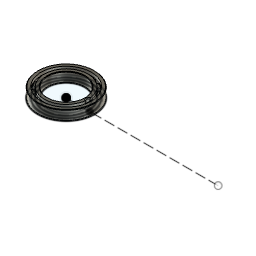
id15 bearing v6 (Autodesk Fusion 360 design; units mm, degrees)
Autodesk Fusion 360 part; units mm, degrees
sketch "Sketch1" plane through (0, 0, 0) normal (0, 0, 1) x (1, 0, 0)
  circle A0 centre (0, 0) radius 7.6
  circle A1 centre (0, 0) radius 8.6 construction
  line L0 (0, 0) -> (62.2874, 0) construction
  circle A2 centre (9.6, 0) radius 1 construction
  circle A3 centre (0, 0) radius 10.6 construction
  circle A4 centre (0, 0) radius 11.6
  circle A5 centre (9.6, 0) radius 0.5 construction
  circle A6 centre (0, 0) radius 9.1
  circle A7 centre (0, 0) radius 10.1
  circle A8 centre (0, 0) radius 8.94
  circle A9 centre (0, 0) radius 10.26
  dimension "d1" = 15.2
  dimension "d2" = 1
  dimension "d3" = 2
  dimension "d4" = 1
  dimension "d5" = 1
  dimension "d6" = -0.16
  dimension "d7" = 0.16
  constraint coincident A0.centre A1.centre
  constraint horizontal L0
  constraint coincident L0 A2.centre
  constraint tangent A1 A2
  constraint concentric A1 A3
  constraint tangent A2 A3
  constraint concentric A0 A4
  constraint concentric A2 A5
  constraint concentric A3 A6
  constraint tangent A5 A6
  constraint concentric A1 A7
  constraint tangent A5 A7
  measures "d1" diameter of A0
  measures "d2" distance of A0 A1
  measures "d3" diameter of A2
  measures "d4" distance of A3 A4
  measures "d5" diameter of A5
extrude "Extrude1" add sketch "Sketch1" along normal blind 4 makes body 1 at (8.9289, -0.4456, 2.6667) makes body 2 at (10.0874, -0.5034, 2.6667) makes body 3 at (11.5856, -0.5782, 2.6667)
sketch "Sketch2" plane through (0, 0, 0) normal (0, 1, 0) x (1, 0, 0)
  line L0 (7.6, 0) -> (7.6, -4) construction
  line L1 (-7.6, -4) -> (-7.6, 0)
  line L2 (9.1, 0) -> (9.1, -4)
  line L3 (-9.1, -4) -> (-9.1, 0)
  line L4 (10.26, 0) -> (10.26, -4) construction
  line L5 (-10.26, -4) -> (-10.26, 0)
  line L6 (8.94, -4) -> (8.94, 0) construction
  line L7 (-8.94, 0) -> (-8.94, -4)
  line L8 (10.1, -4) -> (10.1, 0)
  line L9 (-10.1, 0) -> (-10.1, -4)
  line L10 (11.6, -4) -> (11.6, 0) construction
  line L11 (-11.6, 0) -> (-11.6, -4)
  line L12 (-8.94, -4) -> (-7.6, -4)
  line L13 (7.6, -4) -> (8.94, -4) construction
  line L14 (-10.1, -4) -> (-9.1, -4)
  line L15 (9.1, -4) -> (10.1, -4)
  line L16 (-11.6, -4) -> (-10.26, -4)
  line L17 (10.26, -4) -> (11.6, -4) construction
  line L18 (8.94, 0) -> (7.6, 0) construction
  line L19 (-7.6, 0) -> (-8.94, 0)
  line L20 (10.1, 0) -> (9.1, 0)
  line L21 (-9.1, 0) -> (-10.1, 0)
  line L22 (11.6, 0) -> (10.26, 0) construction
  line L23 (-10.26, 0) -> (-11.6, 0)
  line L24 (7.6, -2) -> (11.6, -2) construction
  line L25 (9.6, -4) -> (9.6, 0) construction
  point P0 (9.6, -2)
  constraint midpoint L0 L24.start
  constraint midpoint L10 L24.end
  constraint midpoint L15 L25.start
  constraint midpoint L20 L25.end
  constraint midpoint L24 P0
sphere "SpherePrimitive1" add diameter 2.1 placed x (1, 0, 0) y (0, 0, -1) z (0, 1, 0) at (9.5, 0, 2) separate body makes body 4
sketch "Sketch5" plane through (0, 0, 0) normal (0, 1, 0) x (1, 0, 0)
  line L0 (-10.1, -4) -> (-9.1, -4)
  line L1 (9.1, -4) -> (10.1, -4)
  line L2 (10.1, 0) -> (9.1, 0)
  line L3 (-9.1, 0) -> (-10.1, 0)
  line L4 (9.1, -4) -> (9.1, 0)
  line L5 (10.1, 0) -> (10.1, -4)
  line L6 (9.6, -4) -> (9.6, 0) construction
  line L7 (9.6, -2) -> (10.1, -2)
  line L8 (9.1, -2.5) -> (10.1, -2.5)
  dimension "d15" = 0.5
  constraint coincident L1.start L4.start
  constraint coincident L2.end L4.end
  constraint coincident L2.start L5.start
  constraint coincident L1.end L5.end
  constraint midpoint L1 L6.start
  constraint midpoint L2 L6.end
  constraint midpoint L6 L7.start
  constraint midpoint L5 L7.end
  constraint coincident L4 L8.start
  constraint coincident L5 L8.end
  constraint perpendicular L5 L8
  measures "d15" distance of L7.start L8
revolve "Revolve2" cut sketch "Sketch5" angle 360 about axis through (0, 0, 1.75) along (0, 0, 1) contours L1 L4 L5 L8 bodies 2
pattern_circular "C-Pattern2" count 15 over 360 about axis through (0, 0, 1.75) along (0, 0, 1) of "SpherePrimitive1" makes body 5 makes body 6 makes body 7 makes body 8 makes body 9 makes body 10 makes body 11 makes body 12 makes body 13 makes body 14 makes body 15 makes body 16 makes body 17 makes body 18
combine "Combine6" operation cut target body 2 tool bodies 4 5 16 17 7 9 6 10 11 8 14 15 12 13 18 keep tools
sketch "Sketch6" plane through (0, 0, 0) normal (0, 1, 0) x (1, 0, 0)
  circle A0 centre (9.5, -2) radius 1.05
  line L0 (8.94, -4) -> (8.94, 0)
  line L1 (-8.94, 0) -> (-8.94, -4)
  line L2 (10.26, 0) -> (10.26, -4)
  line L3 (-10.26, -4) -> (-10.26, 0)
revolve "Revolve3" cut sketch "Sketch6" angle 360 about axis through (0, 0, 1.75) along (0, 0, 1) contours A0 L2 | A0 L0 bodies 1 3
sketch "Sketch7" plane through (0, 0, 2.5) normal (0, 0, 1) x (-1, 0, 0)
  arc A0 (-9.4973, 3.4369) -> (-8.6109, 2.9432) centre (-8.6787, 3.864) ccw
  arc A1 (-9.4973, 3.4369) -> (-10.0741, 0.7231) centre (0, 0) ccw
  arc A2 (-9.0636, 0.8136) -> (-10.0741, 0.7231) centre (-9.5, 0) ccw
  arc A3 (-8.6109, 2.9432) -> (-9.0636, 0.8136) centre (0, 0) ccw
  circle A4 centre (0, 0) radius 10.1
  circle A5 centre (0, 0) radius 9.1
  arc A6 (-8.6109, -2.9432) -> (-9.4973, -3.4369) centre (-8.6787, -3.864) ccw
  arc A7 (-9.0636, -0.8136) -> (-8.6109, -2.9432) centre (0, 0) ccw
  arc A8 (-10.0741, -0.7231) -> (-9.0636, -0.8136) centre (-9.5, 0) ccw
  arc A9 (-10.0741, -0.7231) -> (-9.4973, -3.4369) centre (0, 0) ccw
  circle A10 centre (-9.5, 0) radius 0.9233
  circle A11 centre (-9.5, 0) radius 1.0233
  dimension "d23" = 0.1
  constraint concentric A2 A10
  constraint coincident A8.start A10
extrude "Extrude2" cut sketch "Sketch7" along normal blind 1.5 contours A3 A5 A7 A10 A11 | A5 A10 bodies 1
chamfer "Chamfer1" distance 0.2 angle 45 4 edges at (-10.815, -4.1947, 4) (-10.815, -4.1947, 0) (-7.0857, 2.7483, 4) (-7.0857, 2.7483, 0) on bodies 1 3
chamfer "Chamfer2" distance 0.3 angle 45 1 edges at (8.4767, 0, 4) on bodies 1
hidden bodies 4 5 6 7 8 9 10 11 12 13 14 15 16 17 18
equation "d4 = d2"
equation "d6 = -d7"
